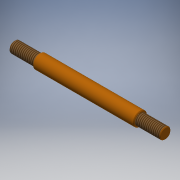
# Autodesk Inventor part: Rear Wheel Axle
Saved by Autodesk Inventor 2018 (Build 220112000, 112)
## iProperties
Created: 2018-08-13
Part Number: Rear Wheel Axle
Material: Generic
Document SubType Name: Modeling
Designer: ruben
Density: 1 g/cm^3
Appearance: Orange
Author: ruben
Autodesk Inventor part; units mm, degrees
ref_plane "YZ Plane" through (0, 0, 0) normal (1, 0, 0) x (0, 1, 0)
ref_plane "XZ Plane" through (0, 0, 0) normal (0, 1, 0) x (-1, 0, 0)
ref_plane "XY Plane" through (0, 0, 0) normal (0, 0, 1) x (1, 0, 0)
sketch "Sketch1" plane through (0, 0, 0) normal (0, 1, 0) x (-1, 0, 0)
  line L0 (1, 0) -> (-6, 0) projected
  line L1 (0, -76.3) -> (0, 76.3) projected
  line L2 (0, -54.5) -> (-4, -54.5)
  line L3 (-4, -54.5) -> (-4, -36.5)
  line L4 (-4, -36.5) -> (-5, -36.5)
  line L5 (-5, -36.5) -> (-5, 36.5)
  line L6 (-5, 36.5) -> (-4, 36.5)
  line L7 (-4, 36.5) -> (-4, 54.5)
  line L8 (-4, 54.5) -> (0, 54.5)
  dimension "d1" = 18
  dimension "d2" = 8
  dimension "d3" = 10
  dimension "d5" = 8
  dimension "d8" = 18
  dimension "d9" = 73
  constraints: 14 end point, 6 perpendicular, 2 point on line, 1 horizontal, 1 other
  measures "d1" distance of L2.end L3.end
  measures "d2" diameter of L3 L1
  measures "d3" diameter of L5 L1
  measures "d5" diameter of L7 L1
  measures "d8" distance of L6.end L7.end
  measures "d9" distance of L4.end L5.end
revolve "Revolution1" add sketch "Sketch1" angle 360 about axis through (0, 0, -10) along (0, 0, 1)
chamfer "Chamfer1" distance 0.5 angle 45 4 edges at (-4, 0, -54.5) (-4, 0, 54.5) (-5, 0, 36.5) (-5, 0, -36.5)
thread "Thread1" size "M8x1.25" class "6g" standard "ANSI Metric M Profile" full length
thread "Thread2" size "M8x1.25" class "6g" standard "ANSI Metric M Profile" full length
equation "\"d5\" = d2"
equation "\"d8\" = d1"
body "Solid1"
